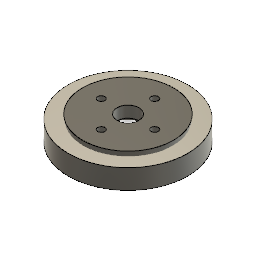
gimbal_bearing_adapter (Autodesk Fusion 360 design; units mm, degrees)
Autodesk Fusion 360 part; units mm, degrees
note: some values were not read from the file. Set by a fixed rule: which sketch regions a step uses.
sketch "Sketch1" plane through (0, 0, 0) normal (0, 1, 0) x (1, 0, 0)
  circle A0 centre (0, 0) radius 15
  circle A1 centre (0, 0) radius 21
  circle A2 centre (0, 0) radius 16
  circle A3 centre (0, 0) radius 3.85
  circle A4 centre (9.4, 0) radius 1.25
  circle A5 centre (0, 9.4) radius 1.25
  circle A6 centre (-9.4, 0) radius 1.25
  circle A7 centre (0, -9.4) radius 1.25
  line L0 (9.4, 0) -> (0, 0) construction
  circle A8 centre (0, 0) radius 15
  line L1 (-4, -21) -> (-21, -21)
  line L2 (-21, -21) -> (-21, -4)
  line L3 (-21, -4) -> (-4, -4)
  line L4 (-4, -4) -> (-4, -21)
  line L5 (4, -21) -> (21, -21)
  line L6 (21, -21) -> (21, -4)
  line L7 (21, -4) -> (4, -4)
  line L8 (4, -4) -> (4, -21)
  line L9 (21, 4) -> (4, 4)
  line L10 (4, 4) -> (4, 21)
  line L11 (4, 21) -> (21, 21)
  line L12 (21, 21) -> (21, 4)
  line L13 (-21, 21) -> (-4, 21)
  line L14 (-4, 21) -> (-4, 4)
  line L15 (-4, 4) -> (-21, 4)
  line L16 (-21, 4) -> (-21, 21)
  line L17 (0, 0) -> (-35.9851, 0)
  line L18 (-35.9851, 0) -> (0, 0) construction
  line L19 (0, -31.769) -> (0, 0) construction
  dimension "d1" = 30
  dimension "d2" = 42
  dimension "d3" = 32
  dimension "d4" = 7.7
  dimension "d5" = 2.5
  dimension "d6" = 9.4
  dimension "d8" = 360
  dimension "d15" = 30
  dimension "d16" = 8
  dimension "d17" = 8
  dimension "d19" = 8
  dimension "d20" = 8
  constraint coincident A0.centre A1.centre
  constraint concentric A1 A2
  constraint concentric A2 A3
  constraint coincident A4.centre L0.start
  constraint horizontal L0
  constraint concentric A2 A8
  constraint horizontal L1
  constraint vertical L2
  constraint horizontal L3
  constraint vertical L4
  constraint horizontal L5
  constraint vertical L6
  constraint horizontal L7
  constraint vertical L8
  constraint horizontal L9
  constraint vertical L10
  constraint horizontal L11
  constraint vertical L12
  constraint horizontal L13
  constraint vertical L14
  constraint horizontal L15
  constraint vertical L16
  constraint collinear L4 L14
  constraint collinear L3 L7
  constraint parallel L0 L17
  constraint parallel L0 L18
  constraint perpendicular L18 L19
  constraint symmetric L4 L8 L19
  constraint symmetric L7 L9 L17
  constraint collinear L2 L16
  constraint collinear L1 L5
  constraint collinear L6 L12
  constraint collinear L11 L13
  constraint tangent A1 L1
  constraint tangent A1 L2
  constraint tangent A1 L12
  constraint tangent A1 L11
  measures "d1" diameter of A0
  measures "d2" diameter of A1
  measures "d3" diameter of A2
  measures "d4" diameter of A3
  measures "d5" diameter of A4
  measures "d6" horizontal distance of A0.centre A4.centre
  measures "d15" diameter of A8
  measures "d16" distance of L3 L15
  measures "d17" distance of L4 L8
  measures "d19" distance of L7 L9
  measures "d20" distance of L10 L14
extrude "Extrude1" add sketch "Sketch1" against normal blind 3.5 contours A0 A8 L3 L4 L7 L8 L9 L10 L14 L15 makes body 1
extrude "Extrude2" add sketch "Sketch1" along normal blind 1.5 and the other way blind 1 contours A0 A8 L3 L4 L7 L8 L9 L10 L14 L15 | A0 A2 A8 L7 L9 | A0 A8 L9 L10 | A0 A2 A8 L9 L10 | A0 A2 A8 L7 L8 | A0 A8 L7 L8 | A0 A2 A8 L10 L14 | A0 A2 A8 L4 L8 | A0 A8 L14 L15 | A0 A2 A8 L14 L15 | A0 A2 A8 L3 L4 | A0 A8 L3 L4 | A0 A2 A8 L15 L17 | A0 A2 A8 L3 L17 bodies 1
extrude "Extrude3" add sketch "Sketch1" against normal blind 7 separate body contours A0 A2 A8 L7 L9 | A0 A2 A8 L9 L10 | A0 A2 A8 L7 L8 | A0 A2 A8 L10 L14 | A1 A2 L7 L9 | A1 A2 L9 L10 | A0 A2 A8 L4 L8 | A1 A2 L7 L8 | A0 A2 A8 L14 L15 | A1 A2 L10 L14 | A0 A2 A8 L3 L4 | A1 A2 L4 L8 | A0 A2 A8 L15 L17 | A1 A2 L14 L15 | A0 A2 A8 L3 L17 | A1 A2 L3 L4 | A1 A2 L15 L17 | A1 A2 L3 L17 makes body 2
fillet "Fillet1" radius 5 4 edges at (-4, -2.25, 4) (4, -2.25, 4) (4, -2.25, -4) (-4, -2.25, -4) on bodies 1
fillet "Fillet1" radius 1.5 8 edges at (-4, -2.25, -14.4568) (4, -2.25, -14.4568) (-14.4568, -2.25, -4) (-14.4568, -2.25, 4) (-4, -2.25, 14.4568) (4, -2.25, 14.4568) (14.4568, -2.25, 4) (14.4568, -2.25, -4) on bodies 1
fillet "Fillet2" radius 1 25 edges at (-14.2239, -3.5, -3.6547) (-11.1332, -3.5, -4) (-5.4645, -3.5, -5.4645) (-4, -3.5, -11.1332) (-3.6547, -3.5, -14.2239) (0, -3.5, -15) (3.6547, -3.5, -14.2239) (4, -3.5, -11.1332) (5.4645, -3.5, -5.4645) (11.1332, -3.5, -4) (14.2239, -3.5, -3.6547) (15, -3.5, 0) (14.2239, -3.5, 3.6547) (11.1332, -3.5, 4) (5.4645, -3.5, 5.4645) (4, -3.5, 11.1332) (3.6547, -3.5, 14.2239) (0, -3.5, 15) (-3.6547, -3.5, 14.2239) (-4, -3.5, 11.1332) (-5.4645, -3.5, 5.4645) (-11.1332, -3.5, 4) (-14.2239, -3.5, 3.6547) (-15, -3.5, 0) (-3.5895, -3.5, 1.3922) on bodies 1
named bodies: "adapter", "bearing"
